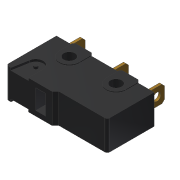
# Autodesk Inventor part: KW-5A-125250V_body#
Saved by Autodesk Inventor 2014 SP2 (Build 180247200, 247)
## iProperties
Created: 2022-06-28
Part Number: KW-5A-125250V_body#
Material: PC_ABS Plastic
Document SubType Name: Modeling
Designer: Воронежский
Mass: 0.399744 g
Surface Area: 9.86977 cm^2
Volume: 1.11888 cm^3
Density: 0.357273 g/cm^3
Appearance: Smooth - Dark Gray
TSKDver: 3.3.4.0
TSKD_DataStamp: 05.07.2022 15:10:27
Login: TAVRIDA\VPO
PCname: S-PC406
ESKDmaterialDescription: -
Company: ООО "Предприятие "Таврида Электрик Украина"
МатериалОбозначениеСтрокой: =<МатериалФорма> <МатериалРазмер>/<Material>
TEL_ID: -
Mass(g): =<Mass>
VLDS_FailCnt: 1
МатериалЕСКД: -
Author: Воронежский
Autodesk Inventor part; units mm, degrees
ref_plane "YZ Plane" through (0, 0, 0) normal (1, 0, 0) x (0, 1, 0)
ref_plane "XZ Plane" through (0, 0, 0) normal (0, 1, 0) x (-1, 0, 0)
ref_plane "XY Plane" through (0, 0, 0) normal (0, 0, 1) x (1, 0, 0)
sketch "Sketch2" plane through (0, 0, 0) normal (0, 0, 1) x (1, 0, 0)
  line L0 (-7, 4.75) -> (12.8, 4.75)
  line L1 (12.8, 4.75) -> (12.8, -4.75)
  line L2 (12.8, -4.75) -> (-7, -4.75)
  line L3 (-7, -4.75) -> (-7, 4.75)
  line L4 (-3.9, 4.75) -> (0.1, 4.75)
  line L5 (0.1, 4.75) -> (0.1, 5.15)
  line L6 (0.1, 5.15) -> (-3.9, 5.15)
  line L7 (-3.9, 5.15) -> (-3.9, 4.75)
  line L8 (5.6, 4.75) -> (9.6, 4.75)
  line L9 (9.6, 4.75) -> (9.6, 5.15)
  line L10 (9.6, 5.15) -> (5.6, 5.15)
  line L11 (5.6, 5.15) -> (5.6, 4.75)
  line L12 (-7, -4.75) -> (3, -4.75)
  line L13 (3, -4.75) -> (3, -5.45)
  line L14 (3, -5.45) -> (-7, -5.45)
  line L15 (-7, -5.45) -> (-7, -4.75)
  circle A0 centre (-1.9, 2.25) radius 1.15
  circle A1 centre (7.6, 2.25) radius 1.15
  point P0 (0, 0)
  dimension "d2" = 19.8
  dimension "d3" = 9.5
  dimension "d4" = 7
  dimension "d5" = 4.75
  dimension "d6" = 0.4
  dimension "d8" = 0.4
  dimension "d10" = 4
  dimension "d11" = 4
  dimension "d13" = 10
  dimension "d14" = 5.1
  dimension "d15" = 9.5
  dimension "d16" = 2
  dimension "d17" = 2
  dimension "d18" = 3.2
  dimension "d21" = 2.3
  dimension "d22" = 2.3
  dimension "d80" = 7.2
  dimension "d81" = 2.5
  dimension "d82" = 2.5
  dimension "d83" = 10.2
  constraints: 32 end point, 8 parallel, 4 horizontal, 4 perpendicular, 2 centre point, 2 coincident, 2 point on line
  measures "d2" distance of L0.start L0.end
  measures "d3" distance of L0.end L1.end
  measures "d4" distance from line of L3 point (0, 0)
  measures "d5" distance from line of L0 point (0, 0)
  measures "d6" distance between parallel lines of L6 L0
  measures "d8" distance of L8.end L9.end
  measures "d10" distance of L5.end L6.end
  measures "d11" distance of L9.end L10.end
  measures "d13" distance of L13.end L14.end
  measures "d14" distance from line of point (-1.9, 2.25) L3
  measures "d15" distance of point (7.6, 2.25) point (-1.9, 2.25)
  measures "d16" distance from line of L7 point (-1.9, 2.25)
  measures "d17" distance from line of L11 point (7.6, 2.25)
  measures "d18" distance between parallel lines of L9 L1
  measures "d21" diameter of A0
  measures "d22" diameter of A1
  measures "d81" distance from line of point (-1.9, 2.25) L4
  measures "d82" distance from line of point (7.6, 2.25) L0
  measures "d83" distance between parallel lines of L14 L0
extrude "Extrusion1" add sketch "Sketch2" along normal mid plane 6
chamfer "Chamfer1" distance 0.4 angle 45 4 edges at (-3.9, 5.15, 0) (0.1, 5.15, 0) (5.6, 5.15, 0) (9.6, 5.15, 0)
chamfer "Chamfer3" distance 0.7 angle 45 1 edges at (3, -5.45, 0)
sketch "Sketch3" plane through (0, 0, 3) normal (0, 0, 1) x (1, 0, 0)
  line L0 (9.2, 5.15) -> (9.6, 4.75) projected
  line L1 (9.6, 5.15) -> (5.6, 5.15) projected
  line L2 (5.6, 4.75) -> (6, 5.15) projected
  line L3 (-0.3, 5.15) -> (0.1, 4.75) projected
  line L4 (0.1, 5.15) -> (-3.9, 5.15) projected
  line L5 (-3.9, 4.75) -> (-3.5, 5.15) projected
  circle A0 centre (7.6, 2.25) radius 1.15 projected
  circle A1 centre (-1.9, 2.25) radius 1.15 projected
  circle A2 centre (-1.9, 2.25) radius 2
  circle A3 centre (7.6, 2.25) radius 2
  line L6 (-3.9, 2.25) -> (-3.9, 4.75)
  line L7 (0.1, 2.25) -> (0.1, 4.75)
  line L8 (5.6, 2.25) -> (5.6, 4.75)
  line L9 (9.6, 2.25) -> (9.6, 4.75)
  point P0 (0, 0)
  dimension "d28" = 4
  dimension "d29" = 4
  dimension "d30" = 4
  constraints: 8 end point, 4 point on circle, 4 tangent, 2 centre point, 2 coincident
  measures "d28" distance of L3.end L5.start
  measures "d29" diameter of A2
  measures "d30" diameter of A3
extrude "Extrusion2" add sketch "Sketch3" along normal blind 0.2
mirror "Mirror1" about plane through (0, 0, 0) normal (0, 0, 1) of "Extrusion2"
sketch "Sketch4" plane through (-7, -5.45, -3) normal (0, -1, 0) x (1, 0, 0)
  line L0 (6, 5) -> (8, 5)
  line L1 (8, 5) -> (8, 1)
  line L2 (8, 1) -> (6, 1)
  line L3 (6, 1) -> (6, 5)
  point P0 (7, 3)
  dimension "d33" = 2
  dimension "d34" = 4
  dimension "d35" = 1
  dimension "d36" = 2
  constraints: 8 end point, 2 parallel, 1 horizontal, 1 perpendicular
  measures "d33" distance of L0.start L0.end
  measures "d34" distance of L2.end L0.start
  measures "d35" distance from line of point (7, 3) L1
  measures "d36" distance from line of L0 point (7, 3)
extrude "Extrusion3" cut sketch "Sketch4" against normal blind 4
sketch "Sketch5" plane through (-7, 4.75, 3) normal (0, 1, 0) x (1, 0, 0)
  line L0 (7.1, 6) -> (12.6, 6)
  line L1 (12.6, 0) -> (7.1, 0)
  line L2 (19.6, 0) -> (16.4, 0)
  line L3 (16.4, 6) -> (19.6, 6)
  line L4 (1.3, 4.7) -> (1.8, 4.7)
  line L5 (1.8, 4.7) -> (1.8, 1.3)
  line L6 (1.8, 1.3) -> (1.3, 1.3)
  line L7 (1.3, 1.3) -> (1.3, 4.7)
  line L8 (10.1, 4.7) -> (10.6, 4.7)
  line L9 (10.6, 4.7) -> (10.6, 1.3)
  line L10 (10.6, 1.3) -> (10.1, 1.3)
  line L11 (10.1, 1.3) -> (10.1, 4.7)
  line L12 (-0.2, 3) -> (19.6, 3) construction
  line L13 (17.4, 4.7) -> (17.9, 4.7)
  line L14 (17.9, 4.7) -> (17.9, 1.3)
  line L15 (17.9, 1.3) -> (17.4, 1.3)
  line L16 (17.4, 1.3) -> (17.4, 4.7)
  line L17 (0, 0) -> (0, 6)
  line L18 (0, 6) -> (3.1, 6)
  line L19 (0, 0) -> (0, 6)
  line L20 (19.8, 0) -> (16.6, 0)
  line L21 (19.8, 6) -> (19.8, 0)
  line L22 (0, 6) -> (3.1, 6)
  line L23 (3.1, 0) -> (3.1, 6)
  line L24 (3.1, 0) -> (0, 0)
  line L25 (12.6, 0) -> (12.6, 6)
  line L26 (7.1, 6) -> (12.6, 6)
  line L27 (7.1, 6) -> (7.1, 0)
  line L28 (12.6, 0) -> (7.1, 0)
  line L29 (16.4, 6) -> (16.4, 0)
  line L30 (3.1, 0) -> (3.1, 6)
  line L31 (3.1, 0) -> (0, 0)
  line L32 (12.6, 0) -> (12.6, 6)
  line L33 (7.1, 6) -> (7.1, 0)
  line L34 (16.6, 6) -> (16.6, 0)
  line L35 (16.6, 6) -> (19.8, 6)
  line L36 (3.1, 0) -> (0.4, 0) projected
  line L37 (1.55, 4.7) -> (1.55, 1.3) construction
  line L38 (10.35, 4.7) -> (10.35, 1.3) construction
  line L39 (17.65, 4.7) -> (17.65, 1.3) construction
  point P0 (7, 3)
  dimension "d39" = 3.4
  dimension "d40" = 3.4
  dimension "d41" = 0.5
  dimension "d42" = 0.5
  dimension "d43" = 1.7
  dimension "d44" = 1.7
  dimension "d46" = 9.3
  dimension "d47" = 3.4
  dimension "d48" = 0.5
  dimension "d49" = 1.7
  dimension "d50" = 16.6
  dimension "d87" = 8.8
  dimension "d88" = 7.3
  dimension "d89" = 3.1
  dimension "d90" = 1.55
  dimension "d91" = 6
  dimension "d92" = 3
  constraints: 78 end point, 6 midpoint, 6 parallel, 3 horizontal, 3 perpendicular
  measures "d39" distance of L6.end L4.start
  measures "d40" distance of L10.end L8.start
  measures "d41" distance of L4.start L4.end
  measures "d42" distance of L8.start L8.end
  measures "d43" distance between parallel lines of L4 L12
  measures "d44" distance between parallel lines of L12 L8
  measures "d46" distance between parallel lines of L9 L7
  measures "d47" distance of L13.end L14.end
  measures "d48" distance of L14.end L15.end
  measures "d49" distance between parallel lines of L13 L12
  measures "d50" distance between parallel lines of L14 L7
  measures "d87" distance between parallel lines of L38 L37
  measures "d88" distance between parallel lines of L39 L38
  measures "d89" distance between parallel lines of L17 L23
  measures "d90" distance between parallel lines of L37 L17
  measures "d91" distance between parallel lines of L36 L18
  measures "d92" distance between parallel lines of L12 L18
extrude "Extrusion4" add sketch "Sketch5" along normal blind 4 contours L4 L5 L6 L7 | L8 L9 L10 L11 | L13 L14 L15 L16
chamfer "Chamfer2" distance 0.5 angle 45 6 edges at (-5.45, 8.75, 1.7) (-5.45, 8.75, -1.7) (3.35, 8.75, -1.7) (3.35, 8.75, 1.7) (10.65, 8.75, -1.7) (10.65, 8.75, 1.7)
sketch "Sketch6" plane through (-5.7, 4.75, -1.7) normal (-1, 0, 0) x (0, 0, 1)
  line L0 (0, 0) -> (0, 3.5) projected
  line L1 (3.4, 0) -> (3.4, 3.5) projected
  line L2 (0.5, 4) -> (2.9, 4) projected
  point P0 (1.7, -4.75)
  point P1 (1.7, 2.5)
  dimension "d56" = 3.4
  dimension "d57" = 1.7
  dimension "d58" = 1.5
  measures "d56" distance between parallel lines of L1 L0
  measures "d57" distance from line of point (1.7, 2.5) L0
  measures "d58" distance from line of point (1.7, 2.5) L2
hole "Hole1" at (-5.7, 7.25, 0) direction (1, 0, 0) diameter 1.6 end through all
sketch "Sketch7" plane through (0, 0, 3) normal (0, 0, 1) x (1, 0, 0)
  line L0 (-7, 4.75) -> (-7, -5.45) projected
  line L1 (-7, -5.45) -> (3, -5.45) projected
  line L2 (-4, -5.45) -> (-4, -2.45) construction
  line L3 (-5.5, -5.45) -> (-5.5, -2.45)
  line L4 (-2.5, -2.45) -> (-2.5, -5.45)
  arc A0 (-5.5, -5.45) -> (-2.5, -5.45) centre (-4, -5.45) ccw
  arc A1 (-2.5, -2.45) -> (-5.5, -2.45) centre (-4, -2.45) ccw
  point P0 (2.6, -5.45)
  point P1 (0, 0)
  point P2 (-4, -3.95)
  dimension "d66" = 3
  dimension "d68" = 3
  dimension "d69" = 3
  constraints: 8 end point, 4 point on circle, 4 tangent, 2 centre point, 1 midpoint, 1 parallel, 1 perpendicular, 1 point on line
  measures "d66" distance between parallel lines of L4 L3
  measures "d68" distance between parallel lines of L2 L0
  measures "d69" distance from line of L2.end L1
extrude "Extrusion5" cut sketch "Sketch7" against normal blind 0.5
sketch "Sketch8" plane through (0, 0, 2.5) normal (0, 0, 1) x (1, 0, 0)
  arc A0 (-2.5, -2.45) -> (-5.5, -2.45) centre (-4, -2.45) ccw projected
  circle A1 centre (-4, -2.45) radius 0.4
  point P0 (0, 0)
  dimension "d72" = 0.8
  constraints: 1 centre point, 1 coincident
  measures "d72" diameter of A1
extrude "Extrusion6" add sketch "Sketch8" along normal up to surface (0.5 mm away)
mirror "Mirror2" about plane through (0, 0, 0) normal (0, 0, 1) of "Extrusion5", "Extrusion6"
sketch "Sketch9" plane through (0, 0, -3) normal (0, 0, -1) x (-1, 0, 0)
  arc A0 (5.5, -2.45) -> (2.5, -2.45) centre (4, -2.45) ccw projected
  line L0 (5.5, -2.45) -> (5.5, -5.45) projected
  line L1 (5.5, -5.45) -> (7, -5.45) projected
  line L2 (6.0521, -5.45) -> (5.4772, -2.1895)
  line L3 (6.0521, -5.45) -> (5.5, -5.45)
  point P0 (0, 0)
  dimension "d75" = 10
  constraints: 4 end point, 1 collinear, 1 point on circle, 1 point on line, 1 tangent
  measures "d75" angle of L2 L0
extrude "Extrusion7" cut sketch "Sketch9" against normal up to surface (0.5 mm away)
mirror "Mirror3" about plane through (0, 0, 0) normal (0, 0, 1) of "Extrusion7"
fillet "Fillet1" radius 0.5 2 edges at (12.8, -4.75, 0) (-7, -5.45, 0)
equation "\"d5\" = 0.5 * d3"
equation "\"d8\" = d6"
equation "\"d11\" = d10"
equation "\"d16\" = 0.5 * d10"
equation "\"d17\" = 0.5 * d11"
equation "\"d22\" = d21"
equation "\"d82\" = d81"
equation "\"d29\" = d28"
equation "\"d30\" = d29"
equation "\"d35\" = 0.5 * d33"
equation "\"d36\" = 0.5 * d34"
equation "\"d40\" = d39"
equation "\"d42\" = d41"
equation "\"d43\" = 0.5 * d39"
equation "\"d44\" = 0.5 * d40"
equation "\"d47\" = d39"
equation "\"d48\" = d41"
equation "\"d49\" = 0.5 * d47"
equation "\"d90\" = 0.5 * d89"
equation "\"d92\" = 0.5 * d91"
equation "\"d57\" = 0.5 * d56"
body "Solid1"
